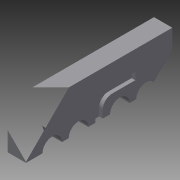
# Autodesk Inventor part: handle
Saved by Autodesk Inventor 2015 (Build 190159000, 159)
## iProperties
Created: 2014-11-04
Part Number: handle
Material: Generic
Document SubType Name: Modeling
Designer: jesse
Density: 1 g/cm^3
Appearance: Default
Author: jesse
Autodesk Inventor part; units mm, degrees
ref_plane "YZ Plane" through (0, 0, 0) normal (1, 0, 0) x (0, 1, 0)
ref_plane "XZ Plane" through (0, 0, 0) normal (0, 1, 0) x (-1, 0, 0)
ref_plane "XY Plane" through (0, 0, 0) normal (0, 0, 1) x (1, 0, 0)
sketch "Sketch1" plane through (0, 0, 0) normal (1, 0, 0) x (0, 1, 0)
  line L0 (0, 0) -> (15.24, 0)
  line L1 (15.24, 0) -> (15.24, -50.8)
  line L2 (15.24, -50.8) -> (0, -50.8)
  arc A0 (0, -12.5154) -> (0, -5.7072) centre (0, -9.1113) ccw
  arc A1 (0, -21.6267) -> (0, -14.8185) centre (0, -18.2226) ccw
  arc A2 (0, -45.0928) -> (0, -38.2846) centre (0, -41.6887) ccw
  arc A3 (0, -35.9815) -> (0, -29.1733) centre (0, -32.5774) ccw
  line L3 (0, -9.1113) -> (5.7639, -9.1113) construction
  line L4 (0, -18.2226) -> (5.7639, -18.2226) construction
  line L5 (0, -32.5774) -> (5.7639, -32.5774) construction
  line L6 (0, -41.6887) -> (5.7639, -41.6887) construction
  line L7 (5.7639, -41.6887) -> (5.7639, -50.8) construction
  line L8 (5.7639, -32.5774) -> (5.7639, -41.6887) construction
  line L9 (5.7639, -18.2226) -> (5.7639, -9.1113) construction
  line L10 (5.7639, -9.1113) -> (5.7639, 0) construction
  line L11 (0, -50.8) -> (0, -45.0928)
  line L12 (0, -38.2846) -> (0, -35.9815)
  line L13 (0, -29.1733) -> (0, -21.6267)
  line L14 (0, -14.8185) -> (0, -12.5154)
  line L15 (0, -5.7072) -> (0, 0)
  dimension "d0" = 15.24
  dimension "d1" = 50.8
  constraints: 32 end point, 8 point on circle, 6 parallel, 5 horizontal, 4 centre point, 4 collinear, 3 equal radius, 3 perpendicular, 3 point on line
  measures "d0" distance of L1.end L2.end
  measures "d1" distance of L0.end L1.end
extrude "Extrusion1" add sketch "Sketch1" along normal blind 6.35
sketch "Sketch2" plane through (6.35, 0, 0) normal (1, 0, 0) x (0, 0, -1)
  line L0 (0, 15.24) -> (0, 0) projected
  line L1 (0, 0) -> (5.7072, 0) projected
  arc A0 (12.5154, 0) -> (5.7072, 0) centre (9.1113, 0) ccw projected
  line L2 (12.5154, 0) -> (14.8185, 0) projected
  arc A1 (21.6267, 0) -> (14.8185, 0) centre (18.2226, 0) ccw projected
  line L3 (21.6267, 0) -> (29.1733, 0) projected
  arc A2 (35.9815, 0) -> (29.1733, 0) centre (32.5774, 0) ccw projected
  line L4 (35.9815, 0) -> (38.2846, 0) projected
  arc A3 (45.0928, 0) -> (38.2846, 0) centre (41.6887, 0) ccw projected
  line L5 (45.0928, 0) -> (50.8, 0) projected
  line L6 (50.8, 0) -> (50.8, 15.24) projected
  line L7 (50.8, 15.24) -> (0, 15.24) projected
  line L8 (21.6267, 0) -> (29.1733, 0) construction
  line L9 (25.4, 0) -> (25.4, 7.1488) construction
  line L10 (25.4, 7.1488) -> (37.9429, 7.1488) construction
  line L11 (37.9429, 5.8788) -> (29.845, 5.8788)
  line L12 (26.67, 2.7038) -> (26.67, 0)
  line L13 (37.9429, 8.4188) -> (24.13, 8.4188)
  line L14 (24.13, 8.4188) -> (24.13, 0)
  line L15 (37.9429, 5.8788) -> (37.9429, 8.4188)
  line L16 (31.3061, 7.1488) -> (31.3061, 8.4188) construction
  line L17 (32.8694, 7.1488) -> (32.8694, 5.8788) construction
  line L18 (24.13, 3.8919) -> (25.4, 3.8919) construction
  line L19 (25.4, 2.7628) -> (26.67, 2.7628) construction
  arc A4 (29.845, 5.8788) -> (26.67, 2.7038) centre (29.845, 2.7038) ccw
  line L20 (24.13, 0) -> (26.67, 0)
  dimension "d4" = 2.54
  dimension "d5" = 3.175
  constraints: 24 end point, 8 point on line, 7 perpendicular, 2 point on circle, 2 tangent, 2 vertical, 1 centre point, 1 collinear, 1 midpoint, 1 parallel, 2 other
  measures "d4" distance of L11.start L13.start
  measures "d5" radius of A4
extrude "Extrusion2" cut sketch "Sketch2" against normal blind 1.27 contours L14 L13 L15 L11 A4 L12 L3
body "Solid1"
